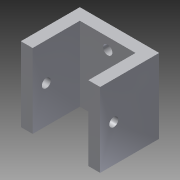
# Autodesk Inventor part: LiftBase2
Saved by Autodesk Inventor 2013 (Build 170138000, 138)
## iProperties
Created: 2013-10-12
Part Number: LiftBase2
Material: Aluminum 6061
Document SubType Name: Modeling
Designer: cobrooks
Density: 1 g/cm^3
Author: cobrooks
Autodesk Inventor part; units mm, degrees
ref_plane "YZ Plane" through (0, 0, 0) normal (1, 0, 0) x (0, 1, 0)
ref_plane "XZ Plane" through (0, 0, 0) normal (0, 1, 0) x (-1, 0, 0)
ref_plane "XY Plane" through (0, 0, 0) normal (0, 0, 1) x (1, 0, 0)
sketch "Sketch1" plane through (0, 0, 0) normal (0, 0, 1) x (1, 0, 0)
  line L0 (0, 0) -> (-42.672, 0)
  line L1 (-42.672, 0) -> (-42.672, 40)
  line L2 (-42.672, 40) -> (0, 40)
  line L3 (0, 40) -> (0, 0)
  dimension "d0" = 42.672
  dimension "d1" = 40
  constraints: 8 end point, 2 parallel, 1 horizontal, 1 perpendicular
  measures "d0" distance of L1.end L2.end
  measures "d1" distance between parallel lines of L0 L2
extrude "Extrusion1" add sketch "Sketch1" along normal blind 6.35
sketch "Sketch2" plane through (0, 0, 6.35) normal (0, 0, 1) x (1, 0, 0)
  line L0 (-42.672, 0) -> (0, 0) projected
  line L1 (-42.672, 40) -> (-36.322, 40)
  line L2 (-36.322, 40) -> (-36.322, 0)
  line L3 (-36.322, 0) -> (-42.672, 0)
  line L4 (-42.672, 0) -> (-42.672, 40)
  dimension "d4" = 6.35
  constraints: 8 end point, 2 parallel, 1 horizontal, 1 perpendicular, 1 point on line
  measures "d4" distance of L2.end L3.end
extrude "Extrusion2" add sketch "Sketch2" along normal blind 25.4
sketch "Sketch3" plane through (0, 0, 6.35) normal (0, 0, 1) x (1, 0, 0)
  line L0 (-36.322, 0) -> (0, 0) projected
  line L1 (0, 40) -> (-6.35, 40)
  line L2 (-6.35, 40) -> (-6.35, 0)
  line L3 (-6.35, 0) -> (0, 0)
  line L4 (0, 0) -> (0, 40)
  dimension "d7" = 6.35
  constraints: 8 end point, 2 parallel, 1 horizontal, 1 perpendicular, 1 point on line
  measures "d7" distance of L3.end L2.end
extrude "Extrusion3" add sketch "Sketch3" along normal blind 25.4
sketch "Sketch4" plane through (0, 0, 0) normal (1, 0, 0) x (0, 0, -1)
  circle A0 centre (-24.4119, 20) radius 2.413
  dimension "d10" = 4.826
  constraints: 1 centre point
  measures "d10" diameter of A0
extrude "Extrusion4" cut sketch "Sketch4" against normal blind 76.2
sketch "Sketch5" plane through (0, 0, 6.35) normal (0, 0, 1) x (1, 0, 0)
  line L0 (-6.35, 40) -> (-36.322, 40) projected
  line L1 (-36.322, 0) -> (-6.35, 0) projected
  point P0 (0, 0)
  point P1 (-21.336, 33.904)
  point P2 (-21.336, 6.096)
  dimension "d13" = 6.096
  dimension "d14" = 6.096
  measures "d13" distance from line of L0 point (-21.336, 33.904)
  measures "d14" distance from line of point (-21.336, 6.096) L1
hole "Hole1" at (-21.336, 33.904, 6.35) at (-21.336, 6.096, 6.35) direction (0, 0, -1) diameter 5 end through all
body "Solid1"
